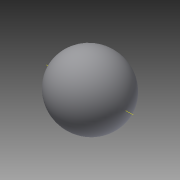
# Autodesk Inventor part: sphere_example
Saved by Autodesk Inventor 2015 (Build 190159000, 159)
## iProperties
Created: 2015-02-06
Part Number: sphere_example
Material: Generic
Document SubType Name: Modeling
Designer: admin
Density: 1 g/cm^3
Appearance: Default
Author: admin
Autodesk Inventor part; units mm, degrees
ref_plane "YZ Plane" through (0, 0, 0) normal (1, 0, 0) x (0, 1, 0)
ref_plane "XZ Plane" through (0, 0, 0) normal (0, 1, 0) x (-1, 0, 0)
ref_plane "XY Plane" through (0, 0, 0) normal (0, 0, 1) x (1, 0, 0)
sketch "Sketch1" plane through (0, 0, 0) normal (0, 1, 0) x (-1, 0, 0)
  line L0 (3.9809, 0) -> (-4.0213, 0)
  arc A0 (3.9809, 0) -> (-4.0213, 0) centre (-0.0202, -0.3233) ccw
  line L1 (5.5813, 0) -> (-5.6217, 0) projected
  point P0 (0, 0)
  dimension "d0" = 90
  constraints: 2 end point, 2 point on circle, 1 centre point, 1 horizontal
revolve "Revolution1" add sketch "Sketch1" angle 360 about axis through (-10, 0, 0) along (1, 0, 0)
body "Solid1"
